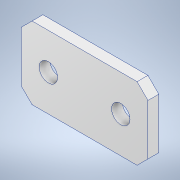
# Autodesk Inventor part: Platinas de unión
Saved by Autodesk Inventor 2020.3 (Build 243373000, 373)
## iProperties
Created: 2021-03-02
Part Number: Platinas de unión
Material: Aluminum 6061
Document SubType Name: Modeling
Designer: juanp
Density: 2.7 g/cm^3
Appearance: Aluminum - Flat
Author: juanp
Autodesk Inventor part; units mm, degrees
ref_plane "YZ Plane" through (0, 0, 0) normal (1, 0, 0) x (0, 1, 0)
ref_plane "XZ Plane" through (0, 0, 0) normal (0, 1, 0) x (-1, 0, 0)
ref_plane "XY Plane" through (0, 0, 0) normal (0, 0, 1) x (1, 0, 0)
sketch "Sketch1" plane through (0, 0, 0) normal (0, 0, 1) x (1, 0, 0)
  line L0 (0, 0) -> (40, 0)
  line L1 (40, 0) -> (40, 20)
  line L2 (40, 20) -> (0, 20)
  line L3 (0, 20) -> (0, 0)
  line L4 (0, 10) -> (10, 10) construction
  line L5 (10, 10) -> (30, 10) construction
  circle A0 centre (10, 10) radius 2.55
  circle A1 centre (30, 10) radius 2.55
  line L6 (37.5, 0) -> (37.5, 20)
  line L7 (2.5, 0) -> (2.5, 20)
  dimension "d0" = 40
  dimension "d1" = 20
  dimension "d2" = 10
  dimension "d3" = 20
  dimension "d4" = 5.1
  dimension "d5" = 5.1
  dimension "d8" = 2.5
  dimension "d9" = 2.5
  constraints: 16 end point, 5 point on line, 3 perpendicular, 2 centre point, 2 coincident, 2 horizontal, 2 parallel, 1 midpoint
  measures "d0" distance of L2.end L1.end
  measures "d1" distance of L1.end L0.end
  measures "d2" distance of L4.start L4.end
  measures "d3" distance of L4.end L5.end
  measures "d4" diameter of A0
  measures "d5" diameter of A1
  measures "d8" distance between parallel lines of L7 L3
  measures "d9" distance between parallel lines of L1 L6
extrude "Extrusion1" add sketch "Sketch1" along normal blind 3 contours L7 L2 L6 L0
chamfer "Chamfer1" distance 3 angle 45 4 edges at (37.5, 0, 1.5) (37.5, 20, 1.5) (2.5, 20, 1.5) (2.5, 0, 1.5)
body "Solid1"
